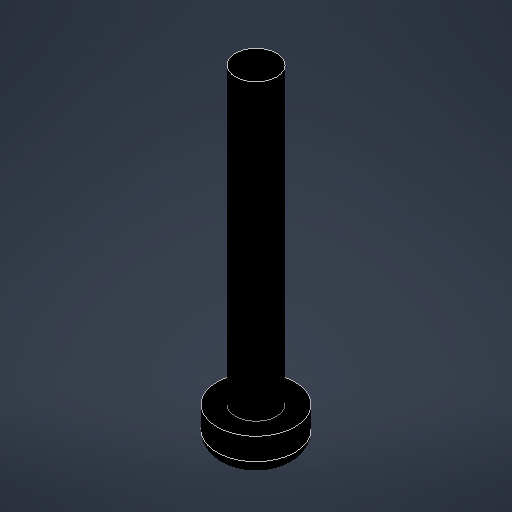
# Autodesk Inventor part: screw
Saved by Autodesk Inventor 2026.2 (Build 302298000, 298)
## iProperties
Created: 2026-01-27
Part Number: screw
Material: Generic
Document SubType Name: Modeling
Designer: test
Density: 1 g/cm^3
Appearance: Default
Author: test
Autodesk Inventor part; units mm, degrees
ref_plane "YZ Plane" through (0, 0, 0) normal (1, 0, 0) x (0, 1, 0)
ref_plane "XZ Plane" through (0, 0, 0) normal (0, 1, 0) x (-1, 0, 0)
ref_plane "XY Plane" through (0, 0, 0) normal (0, 0, 1) x (1, 0, 0)
sketch "Sketch1" plane through (0, 0, 0) normal (0, 0, 1) x (1, 0, 0)
  line L0 (0, 0) -> (1.65, 0)
  line L1 (2.65, 1) -> (2.65, 2.5)
  line L2 (2.65, 2.5) -> (1.4, 2.5)
  line L3 (1.4, 2.5) -> (1.4, 22.5)
  line L4 (1.4, 22.5) -> (0, 22.5)
  line L5 (0, 22.5) -> (0, 0)
  line L6 (0, 0) -> (-1.65, 0)
  line L7 (-2.65, 1) -> (-2.65, 2.5)
  line L8 (-2.65, 2.5) -> (-1.4, 2.5)
  line L9 (-1.4, 2.5) -> (-1.4, 22.5)
  line L10 (-1.4, 22.5) -> (0, 22.5)
  arc A0 (1.65, 0) -> (2.65, 1) centre (1.65, 1) ccw
  arc A1 (-2.65, 1) -> (-1.65, 0) centre (-1.65, 1) ccw
  dimension "d0" = 2.8
  dimension "d1" = 5.3
  dimension "d2" = 1
  dimension "d3" = 2.5
  dimension "d4" = 20
  constraints: 22 end point, 6 symmetric about line, 5 perpendicular, 4 point on circle, 2 centre point, 2 tangent, 1 horizontal, 1 other
  measures "d0" distance between parallel lines of L9 L3
  measures "d1" distance between parallel lines of L1 L7
  measures "d2" radius of A0
  measures "d3" distance between parallel lines of L2 L0
  measures "d4" distance between parallel lines of L2 L4
revolve "Revolution1" add sketch "Sketch1" angle 360 about axis through (0, 22.5, 0) along (0, -1, 0) contours L5 L4 L3 L2 L1 A0 L0
body "Solid1"
